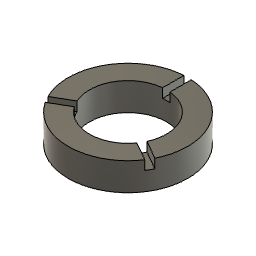
Centering ring 38mm MMT v1 (Autodesk Fusion 360 design; units mm, degrees)
Autodesk Fusion 360 part; units mm, degrees
sketch "Sketch1" plane through (0, 0, 0) normal (0, 1, 0) x (1, 0, 0)
  circle A0 centre (0, 0) radius 20.8
  circle A1 centre (0, 0) radius 32.3
  dimension "d1" = 41.6
  dimension "d2" = 64.6
  constraint coincident A0.centre A1.centre
  measures "d1" diameter of A0
  measures "d2" diameter of A1
extrude "Extrude1" add sketch "Sketch1" along normal blind 10
sketch "Sketch2" plane through (0, 10, 0) normal (0, 1, 0) x (-1, 0, 0)
  circle A0 centre (0, 0) radius 20.8
  circle A1 centre (0, 0) radius 32.3
  line L0 (2, 0) -> (-2, 0)
  line L1 (-2, 0) -> (-2, -41.6)
  line L2 (-2, -41.6) -> (2, -41.6)
  line L3 (2, -41.6) -> (2, 0)
  line L4 (2, 0) -> (-2, -41.6) construction
  line L5 (-2, 0) -> (2, -41.6) construction
  line L6 (1, -1.7321) -> (37.0267, 19.0679)
  line L7 (-1, 1.7321) -> (1, -1.7321)
  line L8 (35.0267, 22.5321) -> (-1, 1.7321)
  line L9 (37.0267, 19.0679) -> (35.0267, 22.5321)
  line L10 (1, -1.7321) -> (35.0267, 22.5321) construction
  line L11 (-1, 1.7321) -> (37.0267, 19.0679) construction
  line L12 (1, 1.7321) -> (-35.0267, 22.5321)
  line L13 (-1, -1.7321) -> (1, 1.7321)
  line L14 (-37.0267, 19.0679) -> (-1, -1.7321)
  line L15 (-35.0267, 22.5321) -> (-37.0267, 19.0679)
  line L16 (1, 1.7321) -> (-37.0267, 19.0679) construction
  line L17 (-1, -1.7321) -> (-35.0267, 22.5321) construction
  point P0 (0, -20.8)
  point P1 (18.0133, 10.4)
  point P2 (-18.0133, 10.4)
  dimension "d5" = 4
  dimension "d7" = 360
  constraint horizontal L0
  constraint perpendicular L0 L1
  constraint parallel L0 L2
  constraint parallel L1 L3
  constraint coincident L4 P0
  constraint coincident L5 P0
  constraint coincident A0 P0
  constraint midpoint A0.centre L0
  measures "d5" distance of L1.end L2.end
extrude "Extrude2" add sketch "Sketch2" along normal blind 5 contours A0 A1 L3 L6 | A0 A1 L8 L12 | A0 A1 L1 L14
